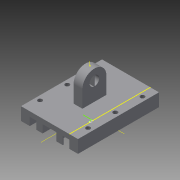
# Autodesk Inventor part: Part2
Saved by Autodesk Inventor 2015 (Build 190159000, 159)
## iProperties
Created: 2016-05-06
Part Number: Part2
Material: Generic
Document SubType Name: Modeling
Designer: Cristi
Density: 1 g/cm^3
Appearance: Default
Author: Cristi
Autodesk Inventor part; units mm, degrees
ref_plane "YZ Plane" through (0, 0, 0) normal (1, 0, 0) x (0, 1, 0)
ref_plane "XZ Plane" through (0, 0, 0) normal (0, 1, 0) x (-1, 0, 0)
ref_plane "XY Plane" through (0, 0, 0) normal (0, 0, 1) x (1, 0, 0)
sketch "Sketch1" plane through (0, 0, 0) normal (0, 0, 1) x (1, 0, 0)
  point P0 (0, 0)
sketch "Sketch2" plane through (0, 0, 0) normal (0, 1, 0) x (-1, 0, 0)
  line L0 (-17.8, 25.3) -> (-17.8, -25.3)
  line L1 (-17.8, -25.3) -> (-12.3, -25.3)
  line L2 (-12.3, -25.3) -> (-12.3, 25.3)
  line L3 (-12.3, 25.3) -> (-17.8, 25.3)
  circle A0 centre (-15, 16.2) radius 1.35
  circle A1 centre (-15, -0.8) radius 1.35
  circle A2 centre (-15, -17.8) radius 1.35
  point P0 (0, 0)
  point P1 (-17.8, 0)
  dimension "d0" = 50.6
  dimension "d1" = 5.5
  dimension "d2" = 2.8
  dimension "d3" = 2.7
  dimension "d4" = 9.1
  dimension "d5" = 2.7
  dimension "d6" = 2.7
  dimension "d7" = 17
  dimension "d8" = 17
  constraints: 8 end point, 3 centre point, 3 perpendicular, 2 vertical alignment, 1 midpoint, 1 vertical
  measures "d0" distance of L0.start L0.end
  measures "d1" distance of L0.end L1.end
  measures "d2" distance from line of L0 A0.centre
  measures "d3" diameter of A0
  measures "d4" distance from line of L3 A0.centre
  measures "d5" diameter of A1
  measures "d6" diameter of A2
  measures "d7" distance of A1.centre A2.centre
  measures "d8" distance of A0.centre A1.centre
extrude "Extrusion1" add sketch "Sketch2" along normal blind 8
sketch "Sketch3" plane through (12.3, 0, -25.3) normal (-1, 0, 0) x (0, 0, 1)
  line L0 (0, 8) -> (50.6, 8)
  line L1 (50.6, 8) -> (0, 8) projected
  line L2 (50.6, 8) -> (50.6, 5)
  line L3 (50.6, 0) -> (50.6, 8) projected
  line L4 (50.6, 5) -> (0, 5)
  line L5 (0, 0) -> (0, 8) projected
  point P0 (25.3, 0)
  dimension "d11" = 3
  constraints: 6 end point, 2 point on line, 1 collinear, 1 perpendicular
  measures "d11" distance of L0.end L2.end
extrude "Extrusion2" add sketch "Sketch3" along normal blind 12.3
mirror "Mirror1" about plane through (0, 0, 0) normal (1, 0, 0) of "Extrusion1", "Extrusion2"
sketch "Sketch4" plane through (0, 8, 0) normal (0, 1, 0) x (1, 0, 0)
  point P0 (0, 0)
sketch "Sketch5" plane through (0, 8, 0) normal (0, 1, 0) x (1, 0, 0)
  line L0 (-2.75, -7.5) -> (-2.75, 7.5)
  line L1 (-2.75, 7.5) -> (2.75, 7.5)
  line L2 (2.75, 7.5) -> (2.75, -7.5)
  line L3 (2.75, -7.5) -> (-2.75, -7.5)
  point P0 (0, 0)
  point P1 (-2.75, 0)
  point P2 (0, 7.5)
  dimension "d14" = 15
  dimension "d15" = 5.5
  constraints: 8 end point, 3 perpendicular, 2 midpoint, 1 horizontal alignment, 1 vertical, 1 vertical alignment
  measures "d14" distance of L0.start L0.end
  measures "d15" distance of L0.end L1.end
extrude "Extrusion3" add sketch "Sketch5" along normal blind 18
sketch "Sketch6" plane through (0, 26, 0) normal (0, 1, 0) x (1, 0, 0)
  point P0 (0, 0)
sketch "Sketch7" plane through (-2.75, 8, -7.5) normal (-1, 0, 0) x (0, 0, 1)
  point P0 (7.5, -8)
sketch "Sketch8" plane through (-2.75, 8, -7.5) normal (-1, 0, 0) x (0, 0, 1)
  circle A0 centre (7.5, 11.35) radius 3
  line L0 (0, 18) -> (15, 18) projected
  point P0 (7.5, -8)
  point P1 (7.5, 18)
  dimension "d18" = 6
  dimension "d19" = 6.65
  constraints: 1 centre point, 1 midpoint, 1 vertical alignment
  measures "d18" diameter of A0
  measures "d19" distance of point (7.5, 18) A0.centre
extrude "Extrusion4" cut sketch "Sketch8" against normal through all
fillet "Fillet1" radius 7.5 1 edges at (0, 26, 7.5)
fillet "Fillet2" radius 7.5 1 edges at (0, 26, -7.5)
sketch "Sketch9" plane through (12.3, 5, -25.3) normal (0, -1, 0) x (1, 0, 0)
  point P0 (-12.3, 25.3)
sketch "Sketch10" plane through (12.3, 5, -25.3) normal (0, -1, 0) x (1, 0, 0)
  line L0 (5.5, 0) -> (-30.1, 0) projected
  line L1 (-4, 0) -> (-8, 0)
  line L2 (-8, 0) -> (-8, 50.6)
  line L3 (0, 50.6) -> (-24.6, 50.6) projected
  line L4 (-4, 50.6) -> (-7.5, 50.6)
  line L5 (-4, 50.6) -> (-4, 50.1)
  line L6 (-4, 50.1) -> (-7.5, 50.1)
  line L7 (-7.5, 0.5) -> (-4, 0.5)
  line L8 (-4, 0.5) -> (-4, 0)
  line L9 (-7.5, 34.7194) -> (-4, 34.7194)
  line L10 (-4, 34.7194) -> (-4, 35.2194)
  line L11 (-4, 35.2194) -> (-7.5, 35.2194)
  line L12 (-7.5, 16.3301) -> (-4, 16.3301)
  line L13 (-4, 16.3301) -> (-4, 15.8301)
  line L14 (-4, 15.8301) -> (-7.5, 15.8301)
  line L15 (-7.5, 15.8301) -> (-7.5, 0.5)
  line L16 (-7.5, 50.1) -> (-7.5, 35.2194)
  line L17 (-7.5, 34.7194) -> (-7.5, 16.3301)
  point P0 (-12.3, 25.3)
  dimension "d24" = 4
  dimension "d25" = 3.5
  dimension "d26" = 0.5
  dimension "d27" = 0.5
  dimension "d28" = 3.5
  dimension "d29" = 0.5
  dimension "d30" = 0.5
  dimension "d33" = 0.5
  dimension "d34" = 0.5
  constraints: 32 end point, 19 perpendicular, 8 point on line, 1 horizontal, 1 vertical
  measures "d24" distance of L1.start L1.end
  measures "d25" distance of L4.start L4.end
  measures "d26" distance of L4.start L5.end
  measures "d27" distance of L7.end L1.start
  measures "d28" distance of L5.end L6.end
  measures "d29" distance of L9.end L10.end
  measures "d30" distance of L12.end L13.end
  measures "d33" distance from line of L2 L7.start
  measures "d34" distance from line of L2 L12.start
extrude "Extrusion5" add sketch "Sketch10" along normal up to surface (5 mm away)
mirror "Mirror2" about plane through (0, 0, 0) normal (1, 0, 0) of "Extrusion5"
sketch "Sketch11" plane through (0, 8, 0) normal (0, 1, 0) x (1, 0, 0)
  line L0 (6.1515, -10.5742) -> (11.6515, -10.5742)
  line L1 (12.3, 25.3) -> (12.3, -25.3) projected
  line L2 (11.6515, -10.5742) -> (11.6515, -12.5742)
  point P0 (0, 0)
  dimension "d35" = 2
  constraints: 4 end point, 2 perpendicular
  measures "d35" distance of L0.end L2.end
sketch "Sketch12" plane through (-2.75, 8, -7.5) normal (-1, 0, 0) x (0, 0, 1)
  point P0 (7.5, -8)
sketch "Sketch14" plane through (2.75, 8, 7.5) normal (1, 0, 0) x (0, 0, -1)
  line L0 (7.25, 14.7235) -> (7.75, 14.7235)
  line L1 (7.75, 14.7235) -> (7.75, 7.9993)
  line L2 (7.75, 7.9993) -> (7.25, 7.9993)
  line L3 (7.25, 7.9993) -> (7.25, 14.7235)
  point P0 (7.5, -8)
  dimension "d40" = 0.5
  constraints: 8 end point, 3 perpendicular, 1 horizontal
  measures "d40" distance of L0.start L0.end
extrude "Extrusion7" add sketch "Sketch14" against normal up to surface (5.5 mm away)
ref_plane "Work Plane1" through (0, 0, 0) normal (1, 0, 0) x (0, 1, 0)
body "Solid1"
